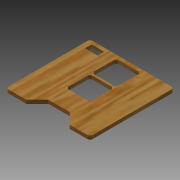
# Autodesk Inventor part: carousel_base
Saved by Autodesk Inventor 2013 (Build 170138000, 138)
## iProperties
Created: 2013-07-24
Part Number: carousel_base
Material: Generic
Document SubType Name: Modeling
Designer: dkboone
Density: 1 g/cm^3
Author: dkboone
Autodesk Inventor part; units mm, degrees
ref_plane "YZ Plane" through (0, 0, 0) normal (1, 0, 0) x (0, 1, 0)
ref_plane "XZ Plane" through (0, 0, 0) normal (0, 1, 0) x (-1, 0, 0)
ref_plane "XY Plane" through (0, 0, 0) normal (0, 0, 1) x (1, 0, 0)
sketch "Sketch1" plane through (0, 0, 0) normal (0, 1, 0) x (-1, 0, 0)
  line L0 (76.2, -76.2) -> (-76.2, -76.2)
  line L1 (-76.2, -76.2) -> (-76.2, 76.2)
  line L2 (76.2, 76.2) -> (76.2, -76.2)
  line L3 (-22.225, -25.4) -> (22.225, -25.4)
  line L4 (22.225, -25.4) -> (22.225, -69.85)
  line L5 (22.225, -69.85) -> (-22.225, -69.85)
  line L6 (-22.225, -69.85) -> (-22.225, -25.4)
  line L7 (-19.05, 56.2) -> (19.05, 56.2)
  line L8 (-76.2, 76.2) -> (-39.05, 76.2)
  line L9 (39.05, 76.2) -> (76.2, 76.2)
  line L10 (19.05, 56.2) -> (39.05, 76.2)
  line L11 (-19.05, 56.2) -> (-39.05, 76.2)
  point P0 (0, 0)
  dimension "d0" = 152.4
  dimension "d2" = 152.4
  dimension "d3" = 76.2
  dimension "d4" = 76.2
  dimension "d5" = 44.45
  dimension "d6" = 44.45
  dimension "d7" = 22.225
  dimension "d26" = 56.2
  dimension "d31" = 45
  dimension "d32" = 45
  dimension "d33" = 38.1
  dimension "d34" = 57.15
  dimension "d56" = 6.35
  constraints: 24 end point, 5 parallel, 3 horizontal, 2 perpendicular, 1 collinear
  measures "d0" distance of L1.end L2.start
  measures "d2" distance of L0.end L1.end
  measures "d3" distance from line of point (0, 0) L1
  measures "d4" distance from line of L0 point (0, 0)
  measures "d5" distance of L3.start L3.end
  measures "d6" distance of L3.end L4.end
  measures "d7" distance from line of point (0, 0) L4
  measures "d26" distance from line of L7 point (0, 0)
  measures "d31" angle of L7 L10
  measures "d32" angle of L7 L11
  measures "d33" distance of L7.start L7.end
  measures "d34" distance from line of L2 L7.end
  measures "d56" distance between parallel lines of L0 L5
extrude "Extrusion1" add sketch "Sketch1" along normal blind 6.35
chamfer "Chamfer2" distance 3.175 angle 45 1 edges at (76.2, 3.175, 76.2)
chamfer "Chamfer3" distance 3.175 angle 45 3 edges at (76.2, 3.175, -76.2) (-76.2, 3.175, -76.2) (-76.2, 3.175, 76.2)
sketch "Sketch3" plane through (0, 6.35, 0) normal (0, 1, 0) x (1, 0, 0)
  line L0 (-18.415, 21.59) -> (18.415, 21.59)
  line L1 (21.59, 18.415) -> (21.59, -18.415)
  line L2 (18.415, -21.59) -> (-18.415, -21.59)
  line L3 (-21.59, -18.415) -> (-21.59, 18.415)
  line L4 (-21.59, 18.415) -> (-18.415, 21.59)
  line L5 (18.415, 21.59) -> (21.59, 18.415)
  line L6 (21.59, -18.415) -> (18.415, -21.59)
  line L7 (-18.415, -21.59) -> (-21.59, -18.415)
  point P0 (0, 0)
  point P1 (-21.59, 21.59)
  point P2 (21.59, -21.59)
  point P3 (21.59, 21.59)
  point P4 (-21.59, -21.59)
  dimension "d41" = 43.18
  dimension "d43" = 43.18
  dimension "d44" = 21.59
  dimension "d45" = 21.59
  dimension "d46" = 3.175
  dimension "d47" = 3.175
  dimension "d48" = 3.175
  dimension "d49" = 3.175
  dimension "d50" = 3.175
  dimension "d51" = 3.175
  dimension "d52" = 3.175
  dimension "d53" = 3.175
  constraints: 16 end point, 8 point on line, 2 parallel, 1 horizontal, 1 perpendicular
  measures "d41" distance of point (-21.59, -21.59) point (-21.59, 21.59)
  measures "d43" distance of point (21.59, -21.59) point (-21.59, -21.59)
  measures "d44" distance from line of point (0, 0) L1
  measures "d45" distance from line of point (0, 0) L0
  measures "d46" distance of L3.end point (-21.59, 21.59)
  measures "d47" distance of L0.start point (-21.59, 21.59)
  measures "d48" distance of L0.end point (21.59, 21.59)
  measures "d49" distance of L1.start point (21.59, 21.59)
  measures "d50" distance of L1.end point (21.59, -21.59)
  measures "d51" distance of L2.start point (21.59, -21.59)
  measures "d52" distance of L2.end point (-21.59, -21.59)
  measures "d53" distance of L3.start point (-21.59, -21.59)
extrude "Extrusion2" cut sketch "Sketch3" against normal through all
chamfer "Chamfer4" distance 3.175 angle 45 4 edges at (-22.225, 3.175, -69.85) (-22.225, 3.175, -25.4) (22.225, 3.175, -69.85) (22.225, 3.175, -25.4)
sketch "Sketch4" plane through (0, 6.35, 0) normal (0, 1, 0) x (1, 0, 0)
  line L0 (73.025, 76.2) -> (-73.025, 76.2) projected
  line L1 (-76.2, 73.025) -> (-76.2, -73.025) projected
  line L2 (-66.675, 69.85) -> (-43.815, 69.85)
  line L3 (-43.815, 69.85) -> (-43.815, 57.785)
  line L4 (-43.815, 57.785) -> (-66.675, 57.785)
  line L5 (-66.675, 57.785) -> (-66.675, 69.85)
  point P0 (0, 0)
  dimension "d60" = 12.065
  dimension "d62" = 22.86
  dimension "d65" = 9.525
  dimension "d66" = 6.35
  constraints: 8 end point, 2 parallel, 1 horizontal, 1 perpendicular
  measures "d60" distance of L4.end L2.start
  measures "d62" distance of L2.start L2.end
  measures "d65" distance between parallel lines of L1 L5
  measures "d66" distance between parallel lines of L0 L2
extrude "Extrusion3" cut sketch "Sketch4" against normal through all
equation "\"d3\" = 0.5 * d0"
equation "\"d4\" = 0.5 * d2"
equation "\"d7\" = 0.5 * d5"
equation "\"d34\" = -0.5 * d33 + 0.5 * d0"
equation "\"d44\" = 0.5 * d43"
equation "\"d45\" = 0.5 * d41"
equation "\"d47\" = d46"
equation "\"d48\" = d46"
equation "\"d49\" = d48"
equation "\"d50\" = d46"
equation "\"d51\" = d50"
equation "\"d52\" = d46"
equation "\"d53\" = d52"
body "Solid1"
